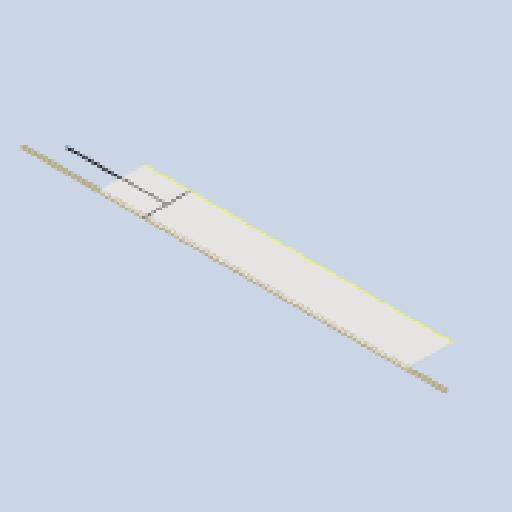
# Autodesk Inventor part: пол2
Saved by Autodesk Inventor 2024.2 (Build 282272000, 272)
## iProperties
Created: 2025-11-16
Part Number: пол2
Material: Типовые
Document SubType Name: Modeling
Designer: katya_notebook
Density: 1 g/cm^3
Appearance: По умолчанию
Author: katya_notebook
Autodesk Inventor part; units mm, degrees
ref_plane "YZ Plane" through (0, 0, 0) normal (1, 0, 0) x (0, 1, 0)
ref_plane "XZ Plane" through (0, 0, 0) normal (0, 1, 0) x (-1, 0, 0)
ref_plane "XY Plane" through (0, 0, 0) normal (0, 0, 1) x (1, 0, 0)
ref_plane "РабПлоскость1" through (1473.2068, -130.4416, 0.2645) normal (0, 1, 0) x (-1, 0, 0)
sketch "Эскиз1" plane through (1473.2068, -130.4416, 0.2645) normal (0, 1, 0) x (-1, 0, 0)
  line L0 (1710.62, 0) -> (1710.62, -242) projected
  line L1 (0, 0) -> (2010.62, 0) projected
  line L2 (100, -242) -> (100, 0) projected
  line L3 (0, -242) -> (2010.62, -242) projected
  line L4 (1710.62, 0) -> (100, 0)
  line L5 (100, 0) -> (100, -242)
  line L6 (100, -242) -> (1710.62, -242)
  line L7 (1710.62, -242) -> (1710.62, 0)
  point P0 (1473.2068, -0.2645)
  constraints: 8 end point, 2 parallel, 1 horizontal, 1 perpendicular
extrude "Выдавливание1" add sketch "Эскиз1" along normal blind 3
sketch "Эскиз2" plane through (1473.2068, -130.4416, 0.2645) normal (0, -1, 0) x (1, 0, 0)
  line L0 (-1473.2068, -0.2645) -> (-1473.2068, -242)
  line L1 (-100, -242) -> (-1710.62, -242) projected
  line L2 (-1473.2068, -121.1323) -> (-1998.2148, -121.1323)
  constraints: 4 end point, 1 horizontal, 1 midpoint, 1 point on line, 1 vertical
